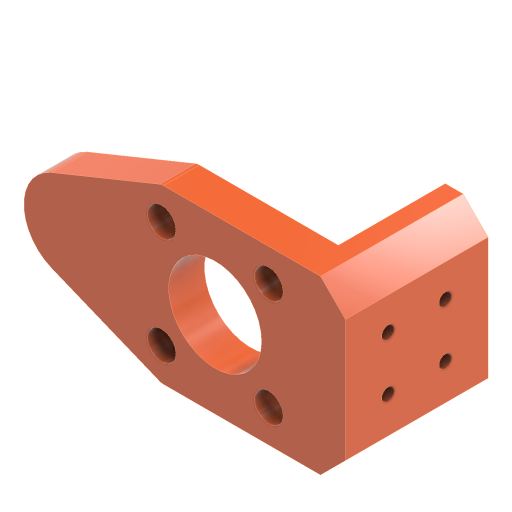
# Autodesk Inventor part: Rear Z Axis Carriage
Saved by Autodesk Inventor 2023.2 (Build 272271000, 271)
## iProperties
Created: 2023-02-17
Part Number: Rear Z Axis Carriage
Material: ABS Plastic
Document SubType Name: Modeling
Designer: remop
Density: 1.06 g/cm^3
Appearance: Smooth - Light Orange
Author: remop
Autodesk Inventor part; units mm, degrees
ref_plane "YZ Plane" through (0, 0, 0) normal (1, 0, 0) x (0, 1, 0)
ref_plane "XZ Plane" through (0, 0, 0) normal (0, 1, 0) x (-1, 0, 0)
ref_plane "XY Plane" through (0, 0, 0) normal (0, 0, 1) x (1, 0, 0)
sketch "Sketch1" plane through (0, 0, 0) normal (0, 0, 1) x (1, 0, 0)
  arc A0 (18.1843, -16.5324) -> (18.7618, -13.101) centre (16.0629, -14.4111) ccw projected
  arc A1 (18.7618, 13.101) -> (18.7618, -13.101) centre (45.75, 0) ccw projected
  arc A2 (18.7618, 13.101) -> (18.1843, 16.5324) centre (16.0629, 14.4111) ccw projected
  line L0 (11.5324, 23.1843) -> (18.1843, 16.5324) projected
  arc A3 (11.5324, 23.1843) -> (8.101, 23.7618) centre (9.4111, 21.0629) ccw projected
  arc A4 (-18.101, 23.7618) -> (8.101, 23.7618) centre (-5, 50.75) ccw projected
  arc A5 (-18.101, 23.7618) -> (-21.5324, 23.1843) centre (-19.4111, 21.0629) ccw projected
  line L1 (-28.1843, 16.5324) -> (-21.5324, 23.1843) projected
  arc A6 (-28.1843, 16.5324) -> (-28.7618, 13.101) centre (-26.0629, 14.4111) ccw projected
  arc A7 (-28.7618, -13.101) -> (-28.7618, 13.101) centre (-55.75, 0) ccw projected
  arc A8 (-28.7618, -13.101) -> (-28.1843, -16.5324) centre (-26.0629, -14.4111) ccw projected
  line L2 (-21.5324, -23.1843) -> (-28.1843, -16.5324) projected
  arc A9 (-21.5324, -23.1843) -> (-18.101, -23.7618) centre (-19.4111, -21.0629) ccw projected
  arc A10 (8.101, -23.7618) -> (-18.101, -23.7618) centre (-5, -50.75) ccw projected
  arc A11 (8.101, -23.7618) -> (11.5324, -23.1843) centre (9.4111, -21.0629) ccw projected
  line L3 (18.1843, -16.5324) -> (11.5324, -23.1843) projected
  circle A12 centre (10, -15) radius 4 projected
  circle A13 centre (-20, -15) radius 4 projected
  circle A14 centre (-20, 15) radius 4 projected
  circle A15 centre (10, 15) radius 4 projected
  circle A16 centre (-5, 0) radius 13 projected
  line L4 (39.4645, -4.5) -> (34.9645, -4.5) projected
  line L5 (34.9645, -4.5) -> (34.9645, 4.5) projected
  line L6 (34.9645, 4.5) -> (39.4645, 4.5) projected
  line L7 (39.4645, 4.5) -> (39.4645, 10) projected
  line L8 (39.4645, 10) -> (31.4645, 10) projected
  line L9 (31.4645, 10) -> (31.4645, -10) projected
  line L10 (31.4645, -10) -> (39.4645, -10) projected
  line L11 (39.4645, -10) -> (39.4645, -4.5) projected
  line L12 (31.4645, -10) -> (31.4645, -17.0711)
  line L13 (31.4645, -17.0711) -> (24.4726, -24.0629)
  line L14 (31.4645, 10) -> (31.4645, 17.0711)
  line L15 (-19.4111, -24.0629) -> (24.4726, -24.0629)
  line L16 (-19.4111, 24.0629) -> (24.4726, 24.0629)
  line L17 (31.4645, 17.0711) -> (24.4726, 24.0629)
  circle A17 centre (-46, 0) radius 12.5
  line L18 (-20.5407, -23.8421) -> (-50.7071, -11.5799)
  line L19 (-50.7071, 11.5799) -> (-20.5407, 23.8421)
  point P0 (0, 0)
  dimension "d0" = 45
  dimension "d1" = 5
  dimension "d4" = 46
  dimension "d5" = 25
  constraints: 16 end point, 8 tangent, 6 point on circle, 3 equal length, 2 vertical, 1 centre point, 1 horizontal alignment, 1 point on line
  measures "d0" angle of L12 L13
  measures "d1" distance from line of L9.end L13
  measures "d4" distance of A17.centre point (0, 0)
  measures "d5" diameter of A17
extrude "Extrusion1" add sketch "Sketch1" along normal blind 10 contours L3 A11 A10 A9 L2 A8 A7 A6 L1 A5 A4 A3 L0 A2 A1 A0 | A0 A1 A2 L0 A3 L16 L17 L14 L9 L12 L13 L15 A11 L3 | L15 A9 A10 A11 | L18 A17 L19 A5 L1 A6 A7 A8 L2 A9 | A3 A4 A5 L16 | A17
sketch "Sketch2" plane through (0, 0, 0) normal (0, 0, -1) x (-1, 0, 0)
  line L0 (-24.4726, -24.0629) -> (-31.4645, -17.0711) projected
  line L1 (19.4111, -24.0629) -> (-24.4726, -24.0629) projected
  arc A0 (19.4111, -24.0629) -> (20.5407, -23.8421) centre (19.4111, -21.0629) ccw projected
  line L2 (50.7071, -11.5799) -> (20.5407, -23.8421) projected
  arc A1 (50.7071, -11.5799) -> (50.7071, 11.5799) centre (46, 0) ccw projected
  line L3 (20.5407, 23.8421) -> (50.7071, 11.5799) projected
  arc A2 (20.5407, 23.8421) -> (19.4111, 24.0629) centre (19.4111, 21.0629) ccw projected
  line L4 (-24.4726, 24.0629) -> (19.4111, 24.0629) projected
  line L5 (-31.4645, 17.0711) -> (-24.4726, 24.0629) projected
  line L6 (-31.4645, -17.0711) -> (-31.4645, 17.0711) projected
  circle A3 centre (-10, -15) radius 4 projected
  circle A4 centre (20, -15) radius 4 projected
  circle A5 centre (20, 15) radius 4 projected
  circle A6 centre (-10, 15) radius 4 projected
  circle A7 centre (5, 0) radius 13 projected
  line L7 (-31.4645, 17.0711) -> (-23.4645, 17.0711)
  line L8 (-23.4645, 17.0711) -> (-23.4645, -17.0711)
  line L9 (-24.4726, -24.0629) -> (-31.4645, -17.0711) projected
  line L10 (-23.4645, -17.0711) -> (-31.4645, -17.0711)
  line L11 (-23.4645, 17.0711) -> (-19.4726, 21.0629)
  line L12 (-19.4726, 21.0629) -> (-19.4726, 24.0629)
  line L13 (-23.4645, -17.0711) -> (-19.4726, -21.0629)
  line L14 (-19.4726, -21.0629) -> (-19.4726, -24.0629)
  line L15 (19.4111, -24.0629) -> (-24.4726, -24.0629) projected
  point P0 (0, 0)
  dimension "d6" = 8
  dimension "d9" = 3
  constraints: 14 end point, 3 perpendicular, 3 point on line, 2 horizontal, 1 parallel, 1 vertical
  measures "d6" distance of L5.start L7.end
  measures "d9" distance of L11.end L12.end
extrude "Extrusion2" add sketch "Sketch2" along normal blind 29.9 contours L0 L10 L13 L14 L1 | L6 L7 L8 L10 | L5 L4 L12 L11 L7
sketch "Sketch3" plane through (23.4645, -17.0711, 0) normal (-1, 0, 0) x (0, 0, 1)
  line L0 (0, 34.1421) -> (0, 0) projected
  line L1 (0, 34.1421) -> (-29.9, 34.1421) projected
  line L2 (-29.9, 0) -> (-29.9, 34.1421) projected
  line L3 (0, 0) -> (-29.9, 0) projected
  point P0 (0, 17.0711)
  point P1 (-1.95, 25.0158)
  point P2 (-17.95, 25.0158)
  point P3 (-17.95, 10.0158)
  point P4 (-1.95, 10.0158)
  dimension "d10" = 15
  dimension "d11" = 16
  dimension "d12" = 11.95
  constraints: 2 horizontal alignment, 2 vertical alignment
  measures "d10" distance of point (-1.95, 10.016) point (-1.95, 25.016)
  measures "d11" distance of point (-17.95, 25.016) point (-1.95, 25.016)
  measures "d12" distance from line of L2 point (-17.95, 25.016)
hole "Hole1" at (23.4645, 7.9447, -1.95) at (23.4645, 7.9447, -17.95) at (23.4645, -7.0553, -17.95) at (23.4645, -7.0553, -1.95) direction (1, 0, 0) diameter 3.6 end through all counterbore diameter 6.5 counterbore depth 3.4 clearance for "Socket Head Cap Screw DIN EN ISO 4762" size "M3" standard "DIN"
sketch "Sketch4" plane through (0, 0, 0) normal (0, 0, -1) x (-1, 0, 0)
  circle A0 centre (5, 0) radius 13 projected
  circle A1 centre (-10, 15) radius 4 projected
  circle A2 centre (20, 15) radius 4 projected
  circle A3 centre (20, -15) radius 4 projected
  circle A4 centre (-10, -15) radius 4 projected
  line L0 (-19.4726, 24.0629) -> (-19.4726, 21.0629) projected
  line L1 (-19.4726, 21.0629) -> (-23.4645, 17.0711) projected
  line L2 (-23.4645, 17.0711) -> (-23.4645, 10.5447) projected
  line L3 (-23.4645, 10.5447) -> (-23.4645, 5.3447) projected
  line L4 (-23.4645, 5.3447) -> (-23.4645, -4.4553) projected
  line L5 (-23.4645, -4.4553) -> (-23.4645, -9.6553) projected
  line L6 (-23.4645, -9.6553) -> (-23.4645, -17.0711) projected
  line L7 (-23.4645, -17.0711) -> (-19.4726, -21.0629) projected
  line L8 (-19.4726, -21.0629) -> (-19.4726, -24.0629) projected
  line L9 (19.4111, -24.0629) -> (-19.4726, -24.0629) projected
  arc A5 (19.4111, -24.0629) -> (20.5407, -23.8421) centre (19.4111, -21.0629) ccw projected
  line L10 (50.7071, -11.5799) -> (20.5407, -23.8421) projected
  arc A6 (50.7071, -11.5799) -> (50.7071, 11.5799) centre (46, 0) ccw projected
  line L11 (20.5407, 23.8421) -> (50.7071, 11.5799) projected
  arc A7 (20.5407, 23.8421) -> (19.4111, 24.0629) centre (19.4111, 21.0629) ccw projected
  line L12 (-19.4726, 24.0629) -> (19.4111, 24.0629) projected
  line L13 (-19.4726, 21.0629) -> (-15.4807, 17.0711)
  line L14 (-15.4807, 17.0711) -> (-15.4807, -17.0711)
  line L15 (-15.4807, -17.0711) -> (-19.4726, -21.0629)
  line L16 (-23.4645, 17.0711) -> (-19.4726, 21.0629) projected
  point P0 (0, 0)
  constraints: 6 end point, 3 perpendicular, 1 vertical
extrude "Extrusion3" cut sketch "Sketch4" against normal blind 2 contours L13 L14 L15 L7 L6 L5 L4 L3 L2 L1
body "Solid1"
